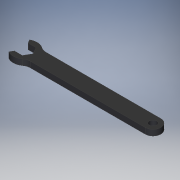
# Autodesk Inventor part: 1pcs-m4-wrench
Saved by Autodesk Inventor 2017 (Build 210142000, 142)
## iProperties
Created: 2018-05-10
Part Number: 1pcs-m4-wrench
Material: Generic
Document SubType Name: Modeling
Designer: ijon
Density: 1 g/cm^3
Appearance: Default
Author: ijon
## iProperties of the stored document 1pcs-m4-wrench_3DPrint.ipt
Created: 2018-05-10
Part Number: 1pcs-m4-wrench_3DPrint
Material: Generic
Document SubType Name: Modeling
Designer: ijon
Density: 1 g/cm^3
Appearance: Default
Author: ijon
Autodesk Inventor part; units mm, degrees
ref_plane "YZ Plane" through (0, 0, 0) normal (1, 0, 0) x (0, 1, 0)
ref_plane "XZ Plane" through (0, 0, 0) normal (0, 1, 0) x (-1, 0, 0)
ref_plane "XY Plane" through (0, 0, 0) normal (0, 0, 1) x (1, 0, 0)
sketch "Sketch1" plane through (0, 0, 0) normal (0, 0, 1) x (1, 0, 0)
  line L0 (1.6454, 2.85) -> (3.2909, 0)
  line L1 (3.2909, 0) -> (1.6454, -2.85)
  line L2 (1.6454, -2.85) -> (-1.6454, -2.85)
  line L3 (-1.6454, -2.85) -> (-1.6498, -2.8425)
  line L4 (-1.6454, 2.85) -> (1.6454, 2.85)
  line L5 (-1.6454, 2.85) -> (-2.5099, 4.3244)
  line L6 (-1.6498, -2.8425) -> (-2.5099, -4.3244)
  line L7 (3.2909, 0) -> (53.2909, 0) construction
  line L8 (5, 0) -> (53.2909, 0) construction
  line L9 (5.3327, -3.25) -> (53.2909, -3.25)
  line L10 (53.2909, 3.25) -> (5.3327, 3.25)
  arc A0 (53.2909, -3.25) -> (53.2909, 3.25) centre (53.2909, 0) ccw
  arc A1 (-2.5099, -4.3244) -> (2.9626, -4.0278) centre (0, 0) ccw
  arc A2 (2.9626, 4.0278) -> (-2.5099, 4.3244) centre (0, 0) ccw
  arc A3 (2.9626, 4.0278) -> (5.3327, 3.25) centre (5.3327, 7.25) ccw
  arc A4 (5.3327, -3.25) -> (2.9626, -4.0278) centre (5.3327, -7.25) ccw
  circle A5 centre (53.2909, 0) radius 1.5
  point P0 (3.7997, 3.25)
  point P1 (29.1454, 0)
  point P2 (3.7997, -3.25)
  dimension "d0" = 5.7
  dimension "d2" = 50
  dimension "d3" = 6.5
  dimension "d4" = 4
  dimension "d5" = 3
  constraints: 24 end point, 12 point on circle, 6 centre point, 6 tangent, 3 coincident, 3 point on line, 1 collinear, 1 equal radius, 1 horizontal, 1 midpoint, 1 parallel, 9 other
  measures "d0" distance between parallel lines of L2 L4
  measures "d2" distance of L0.end L7.end
  measures "d3" diameter of A0
  measures "d4" radius of A3
  measures "d5" diameter of A5
extrude "Extrusion1" add sketch "Sketch1" along normal blind 2.4
body "Solid1"
